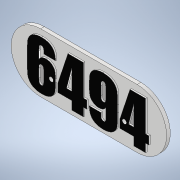
# Autodesk Inventor part: 6494
Saved by Autodesk Inventor 2022 (Build 260153000, 153)
## iProperties
Created: 2021-11-18
Part Number: 6494
Material: Generic
Document SubType Name: Modeling
Designer: TakeHomePC
Density: 1 g/cm^3
Appearance: Default
Author: TakeHomePC
Autodesk Inventor part; units mm, degrees
ref_plane "YZ Plane" through (0, 0, 0) normal (1, 0, 0) x (0, 1, 0)
ref_plane "XZ Plane" through (0, 0, 0) normal (0, 1, 0) x (-1, 0, 0)
ref_plane "XY Plane" through (0, 0, 0) normal (0, 0, 1) x (1, 0, 0)
sketch "Sketch2" plane through (0, 0, 0) normal (0, 0, 1) x (1, 0, 0)
  line L0 (20.8189, 49.0215) -> (188.5216, 49.0215) construction
  line L1 (188.5216, 49.0215) -> (188.5216, -14.4785) construction
  line L2 (188.5216, -14.4785) -> (20.8189, -14.4785) construction
  line L3 (20.8189, -14.4785) -> (20.8189, 49.0215) construction
  line L4 (39.7523, -23.1809) -> (169.7523, -23.1809)
  line L5 (169.7523, 56.3191) -> (39.7523, 56.3191)
  arc A0 (39.7523, 56.3191) -> (39.7523, -23.1809) centre (39.7523, 16.5691) ccw
  arc A1 (169.7523, -23.1809) -> (169.7523, 56.3191) centre (169.7523, 16.5691) ccw
  line L6 (39.7523, 16.5691) -> (169.7523, 16.5691) construction
  line L7 (13.9504, -10.894) -> (193.9504, -10.894)
  line L8 (193.9504, -10.894) -> (193.9504, 37.106)
  line L9 (193.9504, 37.106) -> (13.9504, 37.106)
  line L10 (13.9504, 37.106) -> (13.9504, -10.894)
  line L11 (13.9504, -10.894) -> (193.9504, 37.106) construction
  line L12 (193.9504, -10.894) -> (13.9504, 37.106) construction
  circle A2 centre (55.9046, 6.35) radius 2.85
  circle A3 centre (154.5639, 6.35) radius 2.85
  circle A4 centre (55.9046, 43.9691) radius 4
  circle A5 centre (55.9046, -17.1809) radius 4
  circle A6 centre (154.5639, -17.1809) radius 4
  circle A7 centre (154.5639, 43.9691) radius 4
  line L13 (154.5639, 43.9691) -> (154.5639, -17.1809) construction
  line L14 (55.9046, -17.1809) -> (55.9046, 43.9691) construction
  line L15 (61.6848, 30.8855) -> (45.8457, 30.8855)
  spline S0 degree 2 poles (45.8457, 30.8855) (45.8457, 35.3357) (45.6543, 37.6327) (43.9795, 39.2118) (42.496, 39.2118) knots 0 0 0 1 2 3 3 3
  spline S1 degree 2 poles (42.496, 39.2118) (41.2997, 39.2118) (39.7206, 37.7284) (39.4813, 35.3836) (39.4813, 31.7947) knots 0 0 0 1 2 3 3 3
  line L16 (39.4813, 31.7947) -> (39.4813, 21.65)
  spline S2 degree 2 poles (39.4813, 21.65) (40.6776, 24.234) (45.415, 26.7702) (48.8604, 26.7702) knots 0 0 0 1 2 2 2
  spline S3 degree 2 poles (48.8604, 26.7702) (53.2149, 26.7702) (59.8664, 22.0807) (61.6848, 15.477) (61.6848, 9.8783) knots 0 0 0 1 2 3 3 3
  line L17 (61.6848, 9.8783) -> (61.6848, 4.806)
  spline S4 degree 2 poles (61.6848, 4.806) (61.6848, -1.8455) (60.6799, -8.3534) (56.2296, -13.9043) (48.5254, -16.9668) (43.3574, -16.9668) knots 0 0 0 1 2 3 4 4 4
  spline S5 degree 2 poles (43.3574, -16.9668) (36.993, -16.9668) (28.8103, -13.4258) (24.4079, -6.8221) (23.6422, 0.4993) (23.6422, 11.0268) knots 0 0 0 1 2 3 4 4 4
  line L18 (23.6422, 11.0268) -> (23.6422, 19.7837)
  spline S6 degree 2 poles (23.6422, 19.7837) (23.6422, 31.1247) (24.3122, 38.7811) (29.0974, 45.624) (37.3758, 49.0215) (42.7831, 49.0215) knots 0 0 0 1 2 3 4 4 4
  spline S7 degree 2 poles (42.7831, 49.0215) (49.4346, 49.0215) (58.0002, 44.7148) (61.6848, 36.867) (61.6848, 30.8855) knots 0 0 0 1 2 3 3 3
  spline S8 degree 2 poles (45.8457, 11.0746) (45.8457, 14.4721) (44.3623, 16.9605) (42.6874, 16.9605) knots 0 0 0 1 2 2 2
  spline S9 degree 2 poles (42.6874, 16.9605) (41.0126, 16.9605) (39.4813, 14.5678) (39.4813, 11.0746) knots 0 0 0 1 2 2 2
  line L19 (39.4813, 11.0746) -> (39.4813, -0.4099)
  spline S10 degree 2 poles (39.4813, -0.4099) (39.4813, -4.6209) (40.9169, -7.205) (42.6396, -7.205) knots 0 0 0 1 2 2 2
  spline S11 degree 2 poles (42.6396, -7.205) (43.6445, -7.205) (45.8457, -5.1952) (45.8457, -0.7927) knots 0 0 0 1 2 2 2
  line L20 (45.8457, -0.7927) -> (45.8457, 11.0746)
  line L21 (99.4881, 47.7295) -> (99.4881, 6.2415)
  line L22 (99.4881, 6.2415) -> (103.9862, 6.2415)
  line L23 (103.9862, 6.2415) -> (103.9862, -4.5731)
  line L24 (103.9862, -4.5731) -> (99.4881, -4.5731)
  line L25 (99.4881, -4.5731) -> (99.4881, -15.7705)
  line L26 (99.4881, -15.7705) -> (83.649, -15.7705)
  line L27 (83.649, -15.7705) -> (83.649, -4.5731)
  line L28 (83.649, -4.5731) -> (64.7952, -4.5731)
  line L29 (64.7952, -4.5731) -> (64.7952, 6.2415)
  line L30 (64.7952, 6.2415) -> (78.481, 47.7295)
  line L31 (78.481, 47.7295) -> (99.4881, 47.7295)
  line L32 (83.649, 6.2415) -> (83.649, 33.2781)
  line L33 (83.649, 33.2781) -> (76.6147, 6.2415)
  line L34 (76.6147, 6.2415) -> (83.649, 6.2415)
  line L35 (107.288, 1.1213) -> (123.1272, 1.1213)
  spline S12 degree 2 poles (123.1272, 1.1213) (123.1272, -3.3289) (123.3664, -5.6258) (125.0412, -7.205) (126.5247, -7.205) knots 0 0 0 1 2 3 3 3
  spline S13 degree 2 poles (126.5247, -7.205) (127.721, -7.205) (129.3001, -5.7215) (129.4915, -3.3768) (129.4915, 0.2122) knots 0 0 0 1 2 3 3 3
  line L36 (129.4915, 0.2122) -> (129.4915, 10.3568)
  spline S14 degree 2 poles (129.4915, 10.3568) (128.2952, 7.8207) (123.6057, 5.2366) (120.1125, 5.2366) knots 0 0 0 1 2 2 2
  spline S15 degree 2 poles (120.1125, 5.2366) (115.7579, 5.2366) (109.1064, 9.9262) (107.288, 16.5298) (107.288, 22.1285) knots 0 0 0 1 2 3 3 3
  line L37 (107.288, 22.1285) -> (107.288, 27.2009)
  spline S16 degree 2 poles (107.288, 27.2009) (107.288, 33.8523) (108.3408, 40.3602) (112.7432, 45.9111) (120.4953, 48.9736) (125.6633, 48.9736) knots 0 0 0 1 2 3 4 4 4
  spline S17 degree 2 poles (125.6633, 48.9736) (131.9798, 48.9736) (140.1626, 45.4326) (144.6128, 38.829) (145.3306, 31.5076) (145.3306, 21.0279) knots 0 0 0 1 2 3 4 4 4
  line L38 (145.3306, 21.0279) -> (145.3306, 12.2231)
  spline S18 degree 2 poles (145.3306, 12.2231) (145.3306, 0.8821) (144.7085, -6.7743) (139.8755, -13.6172) (131.6449, -17.0147) (126.2376, -17.0147) knots 0 0 0 1 2 3 4 4 4
  spline S19 degree 2 poles (126.2376, -17.0147) (119.5382, -17.0147) (111.0205, -12.708) (107.288, -4.8602) (107.288, 1.1213) knots 0 0 0 1 2 3 3 3
  spline S20 degree 2 poles (123.1272, 20.9322) (123.1272, 16.9126) (125.2327, 15.0464) (126.3333, 15.0464) knots 0 0 0 1 2 2 2
  spline S21 degree 2 poles (126.3333, 15.0464) (127.9602, 15.0464) (129.4915, 17.439) (129.4915, 20.9322) knots 0 0 0 1 2 2 2
  line L39 (129.4915, 20.9322) -> (129.4915, 32.4168)
  spline S22 degree 2 poles (129.4915, 32.4168) (129.4915, 36.6278) (128.0559, 39.2118) (126.3333, 39.2118) knots 0 0 0 1 2 2 2
  spline S23 degree 2 poles (126.3333, 39.2118) (125.3284, 39.2118) (123.1272, 37.202) (123.1272, 32.7996) knots 0 0 0 1 2 2 2
  line L40 (123.1272, 32.7996) -> (123.1272, 20.9322)
  line L41 (183.1339, 47.7295) -> (183.1339, 6.2415)
  line L42 (183.1339, 6.2415) -> (187.6321, 6.2415)
  line L43 (187.6321, 6.2415) -> (187.6321, -4.5731)
  line L44 (187.6321, -4.5731) -> (183.1339, -4.5731)
  line L45 (183.1339, -4.5731) -> (183.1339, -15.7705)
  line L46 (183.1339, -15.7705) -> (167.2948, -15.7705)
  line L47 (167.2948, -15.7705) -> (167.2948, -4.5731)
  line L48 (167.2948, -4.5731) -> (148.441, -4.5731)
  line L49 (148.441, -4.5731) -> (148.441, 6.2415)
  line L50 (148.441, 6.2415) -> (162.1268, 47.7295)
  line L51 (162.1268, 47.7295) -> (183.1339, 47.7295)
  line L52 (167.2948, 6.2415) -> (167.2948, 33.2781)
  line L53 (167.2948, 33.2781) -> (160.2605, 6.2415)
  line L54 (160.2605, 6.2415) -> (167.2948, 6.2415)
  point P0 (0, 0)
  point P1 (103.9504, 13.106)
  dimension "d33" = 79.5
  dimension "d35" = 130
  dimension "d40" = 63.5
  dimension "d41" = 48
  dimension "d42" = 180
  dimension "d43" = 5.7
  dimension "d44" = 5.7
  dimension "d47" = 8
  constraints: 22 end point, 8 centre point, 4 point on circle, 4 tangent, 3 equal radius, 3 parallel, 3 perpendicular, 2 midpoint, 2 point on line, 1 horizontal, 6 other
  measures "d33" distance between parallel lines of L4 L5
  measures "d35" distance of L6.end L6.start
  measures "d40" distance between parallel lines of L2 L0
  measures "d41" distance of L8.end L7.end
  measures "d42" distance between parallel lines of L8 L10
  measures "d43" diameter of A2
  measures "d44" diameter of A3
  measures "d47" diameter of A4
extrude "Extrusion4" add sketch "Sketch2" along normal blind 2 contours S5 L18 S6 L9 S1 L16 S2 S3 L17 S4 L7 | L7 S4 A5 S5 | S6 S7 A4 L9 S0 S1 | L27 L28 L29 L30 L9 L21 L22 L23 L24 L25 L7 | L7 L25 L26 L27 | S4 A5 | L9 S7 L15 S0 | S7 A4 | S19 L35 S12 S13 L36 S14 S15 L37 S16 L9 S23 L40 S20 S21 L39 S22 S17 L38 S18 L7 | L7 S18 S19 | L30 L31 L21 L9 | L47 L48 L49 L50 L9 L41 L42 L43 L44 L45 L7 | L7 L45 L46 L47 | S16 S17 L9 S22 S23 | L50 L51 L41 L9 | A2 | A3 picked at (53.19, -14.852) picked at (55.598, 43.4971)
extrude "Extrusion7" add sketch "Sketch2" against normal blind 5 from surface at 0 contours A0 L5 A1 L4 | L10 L9 S6 L18 S5 L7 | S5 L18 S6 L9 S1 L16 S2 S3 L17 S4 L7 | L7 S4 A5 S5 | S4 L17 S3 S2 L16 S1 L9 S0 L15 S7 L30 L29 L28 L27 L7 | S6 S7 A4 L9 S0 S1 | L27 L28 L29 L30 L9 L21 L22 L23 L24 L25 L7 | L7 L25 L26 L27 | S4 A5 | A5 S4 | S1 S0 L9 | L25 L24 L23 L22 L21 L9 S16 L37 S15 S14 L36 S13 S12 L35 S19 L7 | L9 S7 L15 S0 | S7 A4 | A4 S7 | S19 L35 S12 S13 L36 S14 S15 L37 S16 L9 S23 L40 S20 S21 L39 S22 S17 L38 S18 L7 | L7 S18 S19 | S18 L38 S17 L9 L50 L49 L48 L47 L7 | L30 L31 L21 L9 | L47 L48 L49 L50 L9 L41 L42 L43 L44 L45 L7 | L7 L45 L46 L47 | L45 L44 L43 L42 L41 L9 L8 L7 | S16 S17 L9 S22 S23 | S23 S22 L9 | L9 S22 L39 S21 S20 L40 S23 | L50 L51 L41 L9 | A6 | A7 | L20 S11 S10 L19 S9 S8 | L34 L33 L32 | L54 L53 L52
extrude "Extrusion9" cut sketch "Sketch2" along normal through all contours A2 | A3
extrude "Extrusion10" cut sketch "Sketch2" along normal blind 3.5 from surface at -5 contours S4 A5 | A5 S4 | S7 A4 | A4 S7 | A6 | A7
chamfer "Chamfer1" distance 3 angle 45 4 edges at (51.9046, 43.9691, -5) (51.9046, -17.1809, -5) (150.5639, 43.9691, -5) (150.5639, -17.1809, -5)
body "Solid3"
